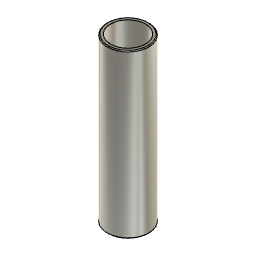
Entretoise_arbre_croix_de_malte_KOSMOS3-0 (Autodesk Fusion 360 design; units mm, degrees)
Autodesk Fusion 360 part; units mm, degrees
sketch "Esquisse1" plane through (0, 0, 0) normal (0, 0, 1) x (1, 0, 0)
  circle A0 centre (0, 0) radius 5
  circle A1 centre (0, 0) radius 4.2
  dimension "d1" = 10
  dimension "d2" = 8.4
  constraint coincident A0.centre A1.centre
  measures "d1" diameter of A0
  measures "d2" diameter of A1
extrude "Extrusion1" add sketch "Esquisse1" along normal blind 39.2
chamfer "Chanfrein1" distance 0.2 angle 45 1 edges at (-4.6616, -1.8081, 39.2)
chamfer "Chanfrein2" distance 0.2 angle 45 1 edges at (-4.6616, -1.8081, 0)
